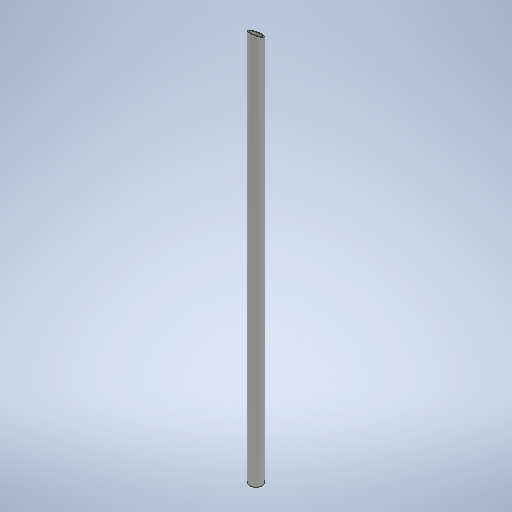
# Autodesk Inventor part: Stainless_Steel_Pipe
Saved by Autodesk Inventor 2026.2 (Build 302298010, 298A)
## iProperties
Created: 2026-05-12
Part Number: Stainless_Steel_Pipe
Material: Generic
Document SubType Name: Modeling
Designer: piete
Density: 1 g/cm^3
Appearance: Stainless - Brushed
Author: piete
Autodesk Inventor part; units mm, degrees
ref_plane "YZ Plane" through (0, 0, 0) normal (1, 0, 0) x (0, 1, 0)
ref_plane "XZ Plane" through (0, 0, 0) normal (0, 1, 0) x (-1, 0, 0)
ref_plane "XY Plane" through (0, 0, 0) normal (0, 0, 1) x (1, 0, 0)
sketch "Sketch1" plane through (0, 0, 0) normal (0, 1, 0) x (-1, 0, 0)
  circle A0 centre (0, 0) radius 4
  circle A1 centre (0, 0) radius 5
  dimension "d0" = 8
  dimension "d1" = 10
  constraints: 2 centre point, 2 coincident
  measures "d0" diameter of A0
  measures "d1" diameter of A1
extrude "Extrusion1" add sketch "Sketch1" along normal blind 330
sketch "Sketch2" plane through (0, 0, 0) normal (1, 0, 0) x (0, 1, 0)
  line L0 (0, -5) -> (330, -5) projected
  line L1 (330, 4) -> (330, -4) projected
  line L2 (330, -5) -> (330, 5) projected
  line L3 (0, -5) -> (0, 5) projected
  line L4 (316, -5) -> (321.7735, 5)
  line L5 (0, 5) -> (330, 5) projected
  line L6 (316, -5) -> (327.547, -5) construction
  line L7 (321.7735, 5) -> (330, 5)
  line L8 (330, 4) -> (0, 4) projected
  line L9 (330, -5) -> (330, 5)
  line L10 (330, -5) -> (316, -5)
  point P0 (0, 0)
  point P1 (321.1962, 4)
  dimension "d4" = 60
  dimension "d5" = 316
  constraints: 10 end point, 2 collinear, 2 point on line, 1 equal length, 1 horizontal, 1 parallel
  measures "d4" angle of L6 L4
  measures "d5" distance from line of L4.start L3
extrude "Extrusion2" cut sketch "Sketch2" along normal through all both and the other way through all contours L4 L8 L1 L2 L0 | L4 L5 L2 L8
body "Solid1"
